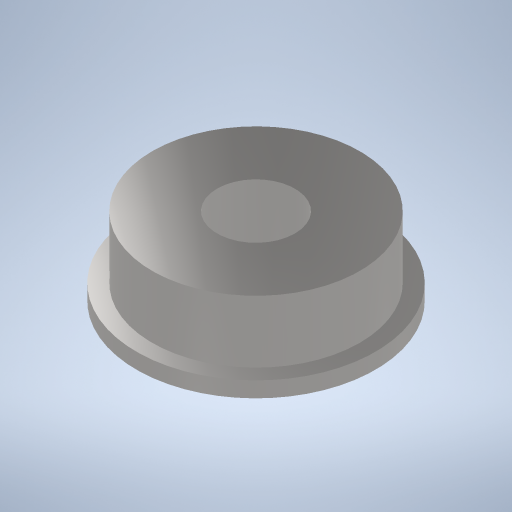
# Autodesk Inventor part: kugellager_drehachse
Saved by Autodesk Inventor 2023 (Build 270158000, 158)
## iProperties
Created: 2022-06-28
Part Number: kugellager_drehachse
Material: Stainless Steel
Document SubType Name: Modeling
Designer: dennis
Density: 8 g/cm^3
Appearance: Semi-Polished
Author: dennis
Autodesk Inventor part; units mm, degrees
ref_plane "YZ Plane" through (0, 0, 0) normal (1, 0, 0) x (0, 1, 0)
ref_plane "XZ Plane" through (0, 0, 0) normal (0, 1, 0) x (-1, 0, 0)
ref_plane "XY Plane" through (0, 0, 0) normal (0, 0, 1) x (1, 0, 0)
sketch "Skizze1" plane through (0, 0, 0) normal (0, 1, 0) x (-1, 0, 0)
  circle A0 centre (0, 0) radius 4.6
  circle A1 centre (0, 0) radius 4
  circle A2 centre (0, 0) radius 1.5
  dimension "d0" = 9.2
  dimension "d1" = 8
  dimension "d2" = 3
  constraints: 3 centre point, 3 coincident
  measures "d0" diameter of A0
  measures "d1" diameter of A1
  measures "d2" diameter of A2
extrude "Extrusion1" add sketch "Skizze1" along normal blind 0.6 contours A0 | A1
extrude "Extrusion2" add sketch "Skizze1" along normal blind 3 contours A1
